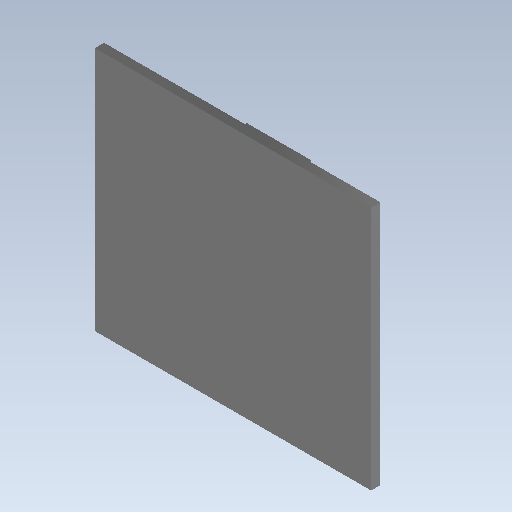
# Autodesk Inventor part: Plate
Saved by Autodesk Inventor 2021.3 (Build 253353000, 353)
## iProperties
Created: 2021-06-01
Part Number: Plate
Material: Wood (Walnut)
Document SubType Name: Modeling
Designer: vivek
Density: 0.55 g/cm^3
Appearance: Walnut - Natural Polished
Author: vivek
Autodesk Inventor part; units mm, degrees
ref_plane "YZ Plane" through (0, 0, 0) normal (1, 0, 0) x (0, 1, 0)
ref_plane "XZ Plane" through (0, 0, 0) normal (0, 1, 0) x (-1, 0, 0)
ref_plane "XY Plane" through (0, 0, 0) normal (0, 0, 1) x (1, 0, 0)
sketch "Sketch1" plane through (0, 0, 0) normal (0, 0, 1) x (1, 0, 0)
  line L0 (150, -133) -> (-150, -133)
  line L1 (-150, -133) -> (-150, 133)
  line L2 (-150, 133) -> (150, 133)
  line L3 (150, 133) -> (150, -133)
  line L4 (0, 0) -> (0, 81.3474)
  line L5 (0, 0) -> (80.8517, 0)
  point P0 (0, 133)
  point P1 (150, 0)
  dimension "d0" = 300
  dimension "d1" = 266
  constraints: 12 end point, 3 parallel, 2 midpoint, 2 perpendicular, 2 point on line, 1 horizontal
  measures "d0" distance of L1.end L2.end
  measures "d1" distance of L0.end L1.end
extrude "Extrusion1" add sketch "Sketch1" along normal blind 10
sketch "Sketch2" plane through (0, 0, 0) normal (0, 0, -1) x (-1, 0, 0)
  line L0 (35, -35) -> (-35, -35)
  line L1 (-35, -35) -> (-35, 35)
  line L2 (-35, 35) -> (35, 35)
  line L3 (35, 35) -> (35, -35)
  line L4 (0, 0) -> (0, 15.9444)
  line L5 (0, 0) -> (16.1389, 0)
  line L6 (35, -95) -> (-35, -95)
  line L7 (-35, -95) -> (-35, -65)
  line L8 (-35, -65) -> (35, -65)
  line L9 (35, -65) -> (35, -95)
  line L10 (35, 65) -> (-35, 65)
  line L11 (-35, 65) -> (-35, 95)
  line L12 (-35, 95) -> (35, 95)
  line L13 (35, 95) -> (35, 65)
  point P0 (0, 35)
  point P1 (35, 0)
  dimension "d4" = 70
  dimension "d7" = 70
  dimension "d8" = 30
  dimension "d9" = 30
  dimension "d10" = 30
  dimension "d11" = 30
  constraints: 28 end point, 7 parallel, 5 perpendicular, 3 collinear, 3 horizontal, 2 midpoint, 2 point on line
  measures "d4" distance of L1.end L2.end
  measures "d7" distance of L7.end L8.end
  measures "d8" distance of L6.end L7.end
  measures "d9" distance of L10.end L11.end
  measures "d10" distance between parallel lines of L2 L10
  measures "d11" distance between parallel lines of L0 L8
extrude "Extrusion2" add sketch "Sketch2" along normal blind 14 contours L0 L1 L2 L3
extrude "Extrusion3" add sketch "Sketch2" along normal blind 40 contours L6 L7 L8 L9 | L10 L11 L12 L13
sketch "Sketch3" plane through (-35, 65, 0) normal (-1, 0, 0) x (0, 0, 1)
  line L0 (0, 30) -> (-40, 30) projected
  line L1 (-40, 0) -> (-40, 30) projected
  circle A0 centre (-20, 15) radius 8
  point P0 (0, -65)
  dimension "d14" = 16
  dimension "d15" = 15
  dimension "d16" = 20
  constraints: 1 centre point
  measures "d14" diameter of A0
  measures "d15" distance from line of L0 A0.centre
  measures "d16" distance from line of L1 A0.centre
extrude "Extrusion4" cut sketch "Sketch3" against normal through all
sketch "Sketch4" plane through (-35, -95, 0) normal (-1, 0, 0) x (0, 0, 1)
  line L0 (0, 30) -> (-40, 30) projected
  line L1 (-40, 0) -> (-40, 30) projected
  circle A0 centre (-20, 15) radius 8
  point P0 (0, 95)
  dimension "d19" = 16
  dimension "d20" = 15
  dimension "d21" = 20
  constraints: 1 centre point
  measures "d19" diameter of A0
  measures "d20" distance from line of L0 A0.centre
  measures "d21" distance from line of L1 A0.centre
extrude "Extrusion5" cut sketch "Sketch4" against normal through all
thread "Thread1" size "M16x2" class "6H" standard "ANSI Metric M Profile" full length
thread "Thread2" size "M16x2" class "6H" standard "ANSI Metric M Profile" full length
body "Solid1"
